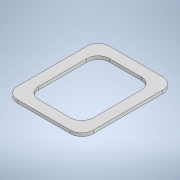
# Autodesk Inventor part: Airpods Pro Top
Saved by Autodesk Inventor 2020 (Build 240168000, 168)
## iProperties
Created: 2020-05-21
Part Number: Airpods Pro Top
Material: Generic
Document SubType Name: Modeling
Designer: maple
Density: 1 g/cm^3
Appearance: Default
Author: maple
Autodesk Inventor part; units mm, degrees
ref_plane "YZ Plane" through (0, 0, 0) normal (1, 0, 0) x (0, 1, 0)
ref_plane "XZ Plane" through (0, 0, 0) normal (0, 1, 0) x (-1, 0, 0)
ref_plane "XY Plane" through (0, 0, 0) normal (0, 0, 1) x (1, 0, 0)
sketch "Sketch1" plane through (0, 0, 0) normal (0, 1, 0) x (-1, 0, 0)
  line L0 (0, 0) -> (13, 0)
  line L1 (13, 0) -> (13, -13)
  line L2 (13, -13) -> (0, -13)
  line L3 (0, -13) -> (0, 0)
  line L4 (13, -13) -> (58.2, -13)
  line L5 (58.2, -13) -> (58.2, -73.6)
  line L6 (58.2, -73.6) -> (13, -73.6)
  line L7 (13, -73.6) -> (13, -13)
  line L8 (58.2, -73.6) -> (71.2, -73.6)
  line L9 (71.2, -73.6) -> (71.2, -86.6)
  line L10 (71.2, -86.6) -> (58.2, -86.6)
  line L11 (58.2, -86.6) -> (58.2, -73.6)
  line L12 (0, 0) -> (71.2, 0)
  line L13 (71.2, 0) -> (71.2, -86.6)
  line L14 (71.2, -86.6) -> (0, -86.6)
  line L15 (0, -86.6) -> (0, 0)
  line L16 (58.2, -13) -> (61.2, -13)
  line L17 (61.2, -13) -> (61.2, -10)
  line L18 (61.2, -10) -> (58.2, -10)
  line L19 (58.2, -10) -> (58.2, -13)
  line L20 (13, -73.6) -> (10, -73.6)
  line L21 (10, -73.6) -> (10, -76.6)
  line L22 (10, -76.6) -> (13, -76.6)
  line L23 (13, -76.6) -> (13, -73.6)
  line L24 (61.2, -10) -> (10, -10)
  line L25 (10, -10) -> (10, -76.6)
  line L26 (10, -76.6) -> (61.2, -76.6)
  line L27 (61.2, -76.6) -> (61.2, -10)
  dimension "d0" = 13
  dimension "d1" = 13
  dimension "d2" = 45.2
  dimension "d3" = 60.6
  dimension "d4" = 13
  dimension "d5" = 13
  dimension "d6" = 3
  dimension "d7" = 3
  dimension "d8" = 3
  dimension "d9" = 3
  constraints: 56 end point, 14 parallel, 7 horizontal, 7 perpendicular
  measures "d0" distance of L1.end L2.end
  measures "d1" distance of L0.end L1.end
  measures "d2" distance of L5.end L6.end
  measures "d3" distance of L4.end L5.end
  measures "d4" distance of L9.end L10.end
  measures "d5" distance of L8.end L9.end
  measures "d6" distance of L18.end L17.end
  measures "d7" distance of L17.end L16.end
  measures "d8" distance of L22.end L21.end
  measures "d9" distance of L21.end L20.end
extrude "Extrusion1" add sketch "Sketch1" along normal blind 3 contours L0 L1 L24 L25 L2 L3 | L12 L13 L8 L27 L17 L18 L24 L1 | L2 L25 L21 L22 L26 L11 L14 L15 | L9 L10 L11 L26 L27 L8
fillet "Fillet1" radius 10.58 4 edges at (0, 1.5, 0) (0, 1.5, -86.6) (-71.2, 1.5, -86.6) (-71.2, 1.5, 0)
fillet "Fillet2" radius 10.58 4 edges at (-61.2, 1.5, -76.6) (-61.2, 1.5, -10) (-10, 1.5, -10) (-10, 1.5, -76.6)
body "Solid1"
